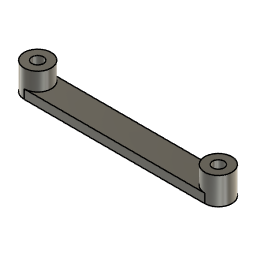
Slider Base v6 (Autodesk Fusion 360 design; units mm, degrees)
Autodesk Fusion 360 part; units mm, degrees
sketch "Sketch1" plane through (0, 0, 0) normal (0, 0, 1) x (1, 0, 0)
  circle A0 centre (0, 0) radius 3.225
  circle A1 centre (100, 0) radius 3.225
  circle A2 centre (0, 0) radius 7.5
  circle A3 centre (100, 0) radius 7.5
  line L0 (100, 7.5) -> (0, 7.5)
  line L1 (0, -7.5) -> (100, -7.5)
  dimension "d3" = 6.45
  dimension "d4" = 6.45
  dimension "d5" = 100
  dimension "d6" = 15
  dimension "d7" = 15
  constraint coincident A0.centre A2.centre
  constraint horizontal A0.centre A1.centre
  constraint concentric A0 A2
  constraint concentric A1 A3
  constraint coincident A3 L0.start
  constraint coincident A2 L0.end
  constraint tangent A2 L0
  constraint coincident A2 L1.start
  constraint coincident A3 L1.end
  constraint tangent A3 L1
  constraint horizontal L1
  constraint tangent A3 L0
  measures "d3" diameter of A0
  measures "d4" diameter of A1
  measures "d5" distance of A0.centre A1.centre
  measures "d6" diameter of A2
  measures "d7" diameter of A3
extrude "Extrude1" add sketch "Sketch1" along normal blind 10 contours A2 | A3 makes body 1 at (7.4627, -0.7468, 3.3333) makes body 2 at (107.4627, -0.7468, 3.3333)
extrude "Extrude2" add sketch "Sketch1" against normal blind 5 contours A0 | A1 | A2 | A2 A3 L0 L1 | A3 bodies 1 2
equation "HoleDiam = 6.45 mm"
equation "SliderDistance = 100 mm"
equation "d3 = HoleDiam"
equation "d4 = HoleDiam"
equation "d5 = SliderDistance"
